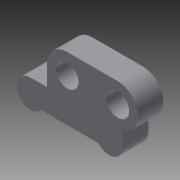
# Autodesk Inventor part: y-motor
Saved by Autodesk Inventor 2015 (Build 190159000, 159)
## iProperties
Created: 2015-04-28
Part Number: y-motor
Material: Generic
Document SubType Name: Modeling
Designer: X
Density: 1 g/cm^3
Appearance: Default
Author: X
Autodesk Inventor part; units mm, degrees
ref_plane "YZ Plane" through (0, 0, 0) normal (1, 0, 0) x (0, 1, 0)
ref_plane "XZ Plane" through (0, 0, 0) normal (0, 1, 0) x (-1, 0, 0)
ref_plane "XY Plane" through (0, 0, 0) normal (0, 0, 1) x (1, 0, 0)
sketch "Sketch1" plane through (0, 0, 0) normal (0, 1, 0) x (-1, 0, 0)
  circle A0 centre (0, 0) radius 8
  circle A1 centre (-20, 0) radius 8
  circle A2 centre (14.5, -13.5) radius 5.5
  circle A3 centre (-16.5, -13.5) radius 5.5
  line L0 (0, 8) -> (-20, 8)
  line L1 (14.5, -8) -> (-16.5, -8)
  line L2 (-12.2574, -17) -> (10.2574, -17)
  line L3 (-22, -13.5) -> (-22, -7.746)
  line L4 (8, 0) -> (8, -8)
  line L5 (0, 0) -> (-25, 0) construction
  dimension "d0" = 16
  dimension "d1" = 11
  dimension "d3" = 9
  dimension "d4" = 20
  dimension "d6" = 2
  dimension "d7" = 31
  constraints: 12 end point, 9 point on circle, 6 tangent, 4 centre point, 2 equal radius, 2 horizontal, 2 perpendicular, 2 point on line, 1 coincident, 1 parallel, 1 vertical
  measures "d0" diameter of A0
  measures "d1" diameter of A2
  measures "d3" distance between parallel lines of L2 L1
  measures "d4" distance of L5.start A1.centre
  measures "d6" distance from line of A1.centre L3
  measures "d7" distance of A3.centre A2.centre
extrude "Extrusion1" add sketch "Sketch1" along normal blind 10
sketch "Sketch3" plane through (0, 10, 0) normal (0, 1, 0) x (1, 0, 0)
  line L0 (0, 0) -> (20, 0) construction
  dimension "d12" = 20
  constraints: 2 coincident, 2 end point, 1 horizontal, 1 point on line
  measures "d12" distance of L0.start point (20, 0)
hole "Hole1" at (0, 10, 0) at (20, 10, 0) direction (0, -1, 0) diameter 9 end through all
body "Solid1"
